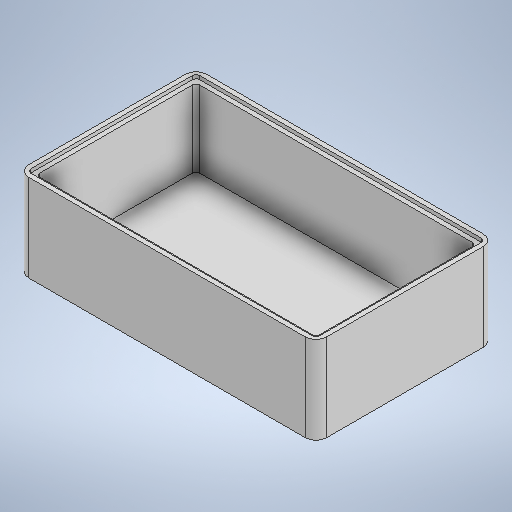
# Autodesk Inventor part: Ver 1
Saved by Autodesk Inventor 2025.2 (Build 292293000, 293)
## iProperties
Created: 2025-05-16
Part Number: Ver 1
Material: Generic
Document SubType Name: Modeling
Designer: CZ
Density: 1 g/cm^3
Appearance: Default
Author: CZ
Autodesk Inventor part; units mm, degrees
ref_plane "YZ Plane" through (0, 0, 0) normal (1, 0, 0) x (0, 1, 0)
ref_plane "XZ Plane" through (0, 0, 0) normal (0, 1, 0) x (-1, 0, 0)
ref_plane "XY Plane" through (0, 0, 0) normal (0, 0, 1) x (1, 0, 0)
sketch "Sketch1" plane through (0, 0, 0) normal (0, 1, 0) x (-1, 0, 0)
  line L0 (-38.5, 22) -> (38.5, 22)
  line L1 (38.5, 22) -> (38.5, -22)
  line L2 (38.5, -22) -> (-38.5, -22)
  line L3 (-38.5, -22) -> (-38.5, 22)
  line L4 (-38.5, 22) -> (38.5, -22) construction
  line L5 (38.5, 22) -> (-38.5, -22) construction
  line L6 (38.5, -22) -> (-38.5, -22)
  line L7 (-38.5, -22) -> (-38.5, 21)
  line L8 (38.5, 21) -> (38.5, -22)
  line L9 (-38, 24.5) -> (38, 24.5)
  line L10 (41, 21.5) -> (41, -21.5)
  line L11 (38, -24.5) -> (-38, -24.5)
  line L12 (-41, -21.5) -> (-41, 21.5)
  line L13 (-41, 24.5) -> (41, -24.5) construction
  line L14 (41, 24.5) -> (-41, -24.5) construction
  arc A0 (41, 21.5) -> (38, 24.5) centre (38, 21.5) ccw
  arc A1 (38, -24.5) -> (41, -21.5) centre (38, -21.5) ccw
  arc A2 (-41, -21.5) -> (-38, -24.5) centre (-38, -21.5) ccw
  arc A3 (-38, 24.5) -> (-41, 21.5) centre (-38, 21.5) ccw
  point P0 (0, 0)
  dimension "d0" = 77
  dimension "d1" = 44
  dimension "d3" = 82
  dimension "d4" = 49
  dimension "d5" = 3
  constraints: 30 end point, 9 point on line, 8 point on circle, 8 tangent, 5 parallel, 4 centre point, 4 midpoint, 3 equal radius, 3 horizontal, 3 perpendicular
  measures "d0" distance of L1.end L2.end
  measures "d1" distance of L0.end L1.end
  measures "d3" distance of L13.end L14.end
  measures "d4" distance of L14.start L13.end
  measures "d5" radius of A0
extrude "Extrusion1" add sketch "Sketch1" along normal blind 2 contours L0 L1 L2 L3 | L9 A0 L10 A1 L11 A2 L12 A3
sketch "Sketch22" plane through (0, 2, 0) normal (0, 1, 0) x (1, 0, 0)
  line L0 (38, 24.5) -> (-38, 24.5) projected
  arc A0 (-38, 24.5) -> (-41, 21.5) centre (-38, 21.5) ccw projected
  line L1 (-41, 21.5) -> (-41, -21.5) projected
  arc A1 (-41, -21.5) -> (-38, -24.5) centre (-38, -21.5) ccw projected
  line L2 (-38, -24.5) -> (38, -24.5) projected
  arc A2 (38, -24.5) -> (41, -21.5) centre (38, -21.5) ccw projected
  line L3 (41, -21.5) -> (41, 21.5) projected
  arc A3 (41, 21.5) -> (38, 24.5) centre (38, 21.5) ccw projected
  line L4 (-38.5, -22) -> (38.5, -22)
  line L5 (38.5, -22) -> (38.5, 22)
  line L6 (38.5, 22) -> (-38.5, 22)
  line L7 (-38.5, 22) -> (-38.5, -22)
  point P0 (0, 0)
  dimension "d80" = 2.5
  dimension "d81" = 2.5
  dimension "d82" = 2.5
  dimension "d83" = 2.5
  constraints: 8 end point, 2 parallel, 1 horizontal, 1 perpendicular
  measures "d80" distance between parallel lines of L0 L6
  measures "d81" distance between parallel lines of L2 L4
  measures "d82" distance between parallel lines of L1 L7
  measures "d83" distance between parallel lines of L3 L5
extrude "Extrusion18" add sketch "Sketch22" along normal blind 22
fillet "Fillet5" radius 1 4 edges at (-38.5, 13, -22) (-38.5, 13, 22) (38.5, 13, 22) (38.5, 13, -22)
sketch "Sketch23" plane through (0, 24, 0) normal (0, 1, 0) x (1, 0, 0)
  line L0 (-38.75, 23.25) -> (38.75, 23.25)
  line L1 (39.75, 22.25) -> (39.75, -22.25)
  line L2 (38.75, -23.25) -> (-38.75, -23.25)
  line L3 (-39.75, -22.25) -> (-39.75, 22.25)
  line L4 (-39.75, 23.25) -> (39.75, -23.25) construction
  line L5 (39.75, 23.25) -> (-39.75, -23.25) construction
  line L6 (41, -21.5) -> (41, 21.5) projected
  line L7 (-38, -24.5) -> (38, -24.5) projected
  line L8 (-38.5, -21) -> (-38.5, 21) projected
  line L9 (-37.5, 22) -> (37.5, 22) projected
  line L10 (38.5, 21) -> (38.5, -21) projected
  line L11 (37.5, -22) -> (-37.5, -22) projected
  arc A0 (-38.5, -21) -> (-37.5, -22) centre (-37.5, -21) ccw projected
  arc A1 (-37.5, 22) -> (-38.5, 21) centre (-37.5, 21) ccw projected
  arc A2 (38.5, 21) -> (37.5, 22) centre (37.5, 21) ccw projected
  arc A3 (37.5, -22) -> (38.5, -21) centre (37.5, -21) ccw projected
  arc A4 (38.75, -23.25) -> (39.75, -22.25) centre (38.75, -22.25) ccw
  arc A5 (39.75, 22.25) -> (38.75, 23.25) centre (38.75, 22.25) ccw
  arc A6 (-38.75, 23.25) -> (-39.75, 22.25) centre (-38.75, 22.25) ccw
  arc A7 (-39.75, -22.25) -> (-38.75, -23.25) centre (-38.75, -22.25) ccw
  point P0 (0, 0)
  dimension "d87" = 1.25
  dimension "d88" = 1.25
  dimension "d91" = 1
  constraints: 12 end point, 8 point on circle, 8 point on line, 8 tangent, 4 centre point, 3 equal radius, 2 midpoint, 2 parallel, 1 horizontal, 1 perpendicular
  measures "d87" distance between parallel lines of L6 L1
  measures "d88" distance between parallel lines of L7 L2
  measures "d91" radius of A4
extrude "Extrusion19" cut sketch "Sketch23" against normal blind 1
body "Solid1"
